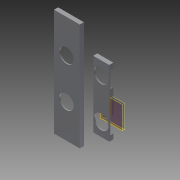
# Autodesk Inventor part: FilterHolder
Saved by Autodesk Inventor 2015 (Build 190159000, 159)
## iProperties
Created: 2015-03-20
Part Number: FilterHolder
Material: NylonD2W
Document SubType Name: Modeling
Designer: Akovo_000
Density: 0.93 g/cm^3
Appearance: Nylon 6
Mass: 9.00848 g
Surface Area: 83.0237 cm^2
Volume: 9.68653 cm^3
Author: Akovo_000
Autodesk Inventor part; units mm, degrees
ref_plane "YZ Plane" through (0, 0, 0) normal (1, 0, 0) x (0, 1, 0)
ref_plane "XZ Plane" through (0, 0, 0) normal (0, 1, 0) x (-1, 0, 0)
ref_plane "Main Work Pane" through (0, 2.75, 7) normal (0, 1, 0) x (-1, 0, 0)
sketch "Panel" plane through (0, 2.75, 7) normal (0, 1, 0) x (-1, 0, 0)
  circle A0 centre (9.0425, 26.1606) radius 11.05 construction
  circle A1 centre (9.0425, -12.8394) radius 11.05 construction
  circle A2 centre (42.8425, -12.8394) radius 11.05
  circle A3 centre (42.8425, 26.1606) radius 11.05
  line L0 (42.8425, -12.8394) -> (42.8425, -12.8394) construction
  line L1 (60.8425, 44.1606) -> (24.8425, 44.1606) construction
  line L2 (24.8425, 44.1606) -> (24.8425, 8.1606) construction
  line L3 (24.8425, 8.1606) -> (60.8425, 8.1606) construction
  line L4 (60.8425, 8.1606) -> (60.8425, 44.1606) construction
  line L5 (60.8425, 44.1606) -> (24.8425, 8.1606) construction
  line L6 (24.8425, 44.1606) -> (60.8425, 8.1606) construction
  line L7 (60.8425, 5.1606) -> (24.8425, 5.1606) construction
  line L8 (24.8425, 5.1606) -> (24.8425, -30.8394) construction
  line L9 (24.8425, -30.8394) -> (60.8425, -30.8394) construction
  line L10 (60.8425, -30.8394) -> (60.8425, 5.1606) construction
  line L11 (60.8425, 5.1606) -> (24.8425, -30.8394) construction
  line L12 (24.8425, 5.1606) -> (60.8425, -30.8394) construction
  line L13 (21.8425, 38.9606) -> (-3.7575, 38.9606) construction
  line L14 (-3.7575, 38.9606) -> (-3.7575, 13.3606) construction
  line L15 (-3.7575, 13.3606) -> (21.8425, 13.3606) construction
  line L16 (21.8425, 13.3606) -> (21.8425, 38.9606) construction
  line L17 (21.8425, 38.9606) -> (-3.7575, 13.3606) construction
  line L18 (-3.7575, 38.9606) -> (21.8425, 13.3606) construction
  line L19 (21.8425, -0.0394) -> (-3.7575, -0.0394) construction
  line L20 (-3.7575, -0.0394) -> (-3.7575, -25.6394) construction
  line L21 (-3.7575, -25.6394) -> (21.8425, -25.6394) construction
  line L22 (21.8425, -25.6394) -> (21.8425, -0.0394) construction
  line L23 (21.8425, -0.0394) -> (-3.7575, -25.6394) construction
  line L24 (-3.7575, -0.0394) -> (21.8425, -25.6394) construction
  line L25 (60.8425, -30.8394) -> (60.8425, 44.1606) construction
  line L26 (60.8425, 44.1606) -> (-3.7575, 44.1606) construction
  line L27 (-3.7575, 44.1606) -> (-3.7575, -30.8394) construction
  line L28 (-3.7575, -30.8394) -> (60.8425, -30.8394) construction
  line L29 (91.5425, -93.8394) -> (-34.4575, -93.8394) construction
  line L30 (-34.4575, -93.8394) -> (-34.4575, 107.1606) construction
  line L31 (-34.4575, 107.1606) -> (91.5425, 107.1606) construction
  line L32 (91.5425, 107.1606) -> (91.5425, -93.8394) construction
  line L33 (42.8425, 15.1106) -> (42.8425, -1.7894) construction
  line L34 (31.7925, 26.1606) -> (20.0925, 26.1606) construction
  line L35 (9.0425, 15.1106) -> (9.0425, -1.7894) construction
  line L36 (20.0925, -12.8394) -> (31.7925, -12.8394) construction
  line L37 (17.4252, 107.1606) -> (17.4252, 44.1606) construction
  line L38 (17.4252, -30.8394) -> (17.4252, -93.8394) construction
  line L39 (60.8425, 6.6606) -> (91.5425, 6.6606) construction
  line L40 (-3.7575, 6.6606) -> (-34.4575, 6.6606) construction
  line L41 (71.3425, 84.9606) -> (89.5425, 84.9606) construction
  line L42 (89.5425, 84.9606) -> (89.5425, 105.1606) construction
  line L43 (89.5425, 105.1606) -> (71.3425, 105.1606) construction
  line L44 (71.3425, 105.1606) -> (71.3425, 84.9606) construction
  line L45 (69.3425, 107.1606) -> (69.3425, 82.9606) construction
  line L46 (69.3425, 82.9606) -> (91.5425, 82.9606) construction
  line L47 (89.5425, -91.8394) -> (71.3425, -91.8394) construction
  line L48 (71.3425, -91.8394) -> (71.3425, -71.6394) construction
  line L49 (71.3425, -71.6394) -> (89.5425, -71.6394) construction
  line L50 (89.5425, -71.6394) -> (89.5425, -91.8394) construction
  line L51 (91.5425, -69.6394) -> (69.3425, -69.6394) construction
  line L52 (69.3425, -69.6394) -> (69.3425, -93.8394) construction
  line L53 (-32.4575, -91.8394) -> (-14.2575, -91.8394) construction
  line L54 (-14.2575, -91.8394) -> (-14.2575, -71.6394) construction
  line L55 (-14.2575, -71.6394) -> (-32.4575, -71.6394) construction
  line L56 (-32.4575, -71.6394) -> (-32.4575, -91.8394) construction
  line L57 (-12.2575, -93.8394) -> (-12.2575, -69.6394) construction
  line L58 (-12.2575, -69.6394) -> (-34.4575, -69.6394) construction
  line L59 (-14.2575, 84.9606) -> (-32.4575, 84.9606) construction
  line L60 (-32.4575, 84.9606) -> (-32.4575, 105.1606) construction
  line L61 (-32.4575, 105.1606) -> (-14.2575, 105.1606) construction
  line L62 (-14.2575, 105.1606) -> (-14.2575, 84.9606) construction
  line L63 (-12.2575, 107.1606) -> (-12.2575, 82.9606) construction
  line L64 (-12.2575, 82.9606) -> (-34.4575, 82.9606) construction
  circle A4 centre (80.4425, 95.0606) radius 2 construction
  line L65 (80.4425, 95.0606) -> (71.3425, 95.0606) construction
  line L66 (80.4425, 95.0606) -> (89.5425, 95.0606) construction
  line L67 (80.4425, 95.0606) -> (80.4425, 105.1606) construction
  line L68 (80.4425, 95.0606) -> (80.4425, 84.9606) construction
  circle A5 centre (-23.3575, 95.0606) radius 2 construction
  line L69 (-23.3575, 95.0606) -> (-23.3575, 84.9606) construction
  line L70 (-23.3575, 95.0606) -> (-23.3575, 105.1606) construction
  line L71 (-23.3575, 95.0606) -> (-32.4575, 95.0606) construction
  line L72 (-23.3575, 95.0606) -> (-14.2575, 95.0606) construction
  circle A6 centre (80.4425, -81.7394) radius 2 construction
  line L73 (80.4425, -81.7394) -> (80.4425, -71.6394) construction
  line L74 (80.4425, -71.6394) -> (80.4425, -81.7394) construction
  line L75 (80.4425, -91.8394) -> (80.4425, -81.7394) construction
  line L76 (80.4425, -81.7394) -> (71.3425, -81.7394) construction
  line L77 (80.4425, -81.7394) -> (89.5425, -81.7394) construction
  circle A7 centre (-23.3575, -81.7394) radius 2 construction
  line L78 (-23.3575, -81.7394) -> (-23.3575, -91.8394) construction
  line L79 (-23.3575, -81.7394) -> (-14.2575, -81.7394) construction
  line L80 (-23.3575, -81.7394) -> (-32.4575, -81.7394) construction
  line L81 (-23.3575, -81.7394) -> (-23.3575, -71.6394) construction
  line L82 (54.9391, 58.7211) -> (29.9084, 58.7211)
  line L83 (29.9084, 58.7211) -> (29.9084, -45.6432)
  line L84 (29.9084, -45.6432) -> (54.9391, -45.6432)
  line L85 (54.9391, -45.6432) -> (54.9391, 58.7211)
  arc A8 (1.229, -20.653) -> (16.856, -20.653) centre (9.0425, -12.8394) ccw
  arc A9 (16.856, -5.0259) -> (1.229, -5.0259) centre (9.0425, -12.8394) ccw
  arc A10 (1.229, 18.347) -> (16.856, 18.347) centre (9.0425, 26.1606) ccw
  arc A11 (16.856, 33.9741) -> (1.229, 33.9741) centre (9.0425, 26.1606) ccw
  line L86 (16.856, -20.653) -> (16.856, -5.0259)
  line L87 (16.856, -5.0259) -> (16.856, 18.347)
  line L88 (16.856, 18.347) -> (16.856, 33.9741)
  line L89 (1.229, 33.9741) -> (1.229, 18.347)
  line L90 (1.229, 18.347) -> (1.229, -5.0259)
  line L91 (1.229, -5.0259) -> (1.229, -20.653)
  line L92 (1.229, -20.653) -> (1.229, -25.6394)
  line L93 (1.229, -25.6394) -> (16.856, -25.6394)
  line L94 (16.856, -25.6394) -> (16.856, -20.653)
  line L95 (16.856, 33.9741) -> (16.856, 38.9606)
  line L96 (16.856, 38.9606) -> (1.229, 38.9606)
  line L97 (1.229, 38.9606) -> (1.229, 33.9741)
  dimension "d337" = 22.1
  dimension "d490" = 36
  dimension "d491" = 36
  dimension "d494" = 3
  dimension "d495" = 25.6
  dimension "d496" = 25.6
  dimension "d497" = 3
  dimension "d498" = 0
  dimension "d582" = 126
  dimension "d583" = 201
  dimension "d584" = 2
  dimension "d585" = 2
  dimension "d586" = 2
  dimension "d587" = 2
  dimension "d588" = 20.2
  dimension "d589" = 18.2
  dimension "d592" = 2
  dimension "d593" = 4
  dimension "d597" = 2
  dimension "d648" = 2
  dimension "d651" = 152.6
  constraints: 196 end point, 27 midpoint, 26 perpendicular, 25 point on line, 23 parallel, 20 equal length, 20 point on circle, 18 collinear, 12 centre point, 11 horizontal, 6 equal radius, 6 line through centre, 6 vertical, 4 coincident
  measures "d337" diameter of A2
  measures "d490" distance of L3.end L2.end
  measures "d491" distance of L2.end L1.end
  measures "d494" distance between parallel lines of L7 L3
  measures "d495" distance of L15.end L14.end
  measures "d496" distance of L14.end L13.end
  measures "d497" distance between parallel lines of L22 L8
  measures "d498" distance between parallel lines of L27 L14
  measures "d582" distance between parallel lines of L30 L32
  measures "d583" distance between parallel lines of L29 L31
  measures "d584" distance between parallel lines of L31 L43
  measures "d585" distance between parallel lines of L32 L42
  measures "d586" distance between parallel lines of L46 L41
  measures "d587" distance between parallel lines of L44 L45
  measures "d588" distance between parallel lines of L41 L43
  measures "d589" distance between parallel lines of L42 L44
  measures "d592" distance between parallel lines of L30 L56
  measures "d593" diameter of A4
  measures "d597" distance between parallel lines of L29 L47
  measures "d648" distance between parallel lines of L62 L63
  measures "d651" distance between parallel lines of L46 L51
ref_plane "Work Plane13" through (0, 2.75, 7) normal (0, -1, 0) x (1, 0, 0)
ref_plane "Work Plane11" through (0, 2.75, 7) normal (0, -1, 0) x (1, 0, 0)
ref_plane "Work Plane12" through (0, 4.75, 7) normal (0, 1, 0) x (1, 0, 0)
extrude "FlatPlane" add sketch "Panel" along normal blind 3 contours L85 L84 L83 L82 | A8 L94 L93 L92 | L90 A10 L87 A9 | L97 L96 L95 A11
sketch "Sketch21" plane through (0, 2.75, 7) normal (0, -1, 0) x (1, 0, 0)
  circle A0 centre (-42.8425, 26.1606) radius 11.05 projected
  circle A1 centre (-42.8425, 26.1606) radius 7
  circle A2 centre (-42.8425, -12.8394) radius 11.05 projected
  circle A3 centre (-42.8425, -12.8394) radius 7
  arc A4 (-1.229, 33.9741) -> (-16.856, 33.9741) centre (-9.0425, 26.1606) ccw projected
  circle A5 centre (-9.0425, 26.1606) radius 7
  arc A6 (-16.856, -20.653) -> (-1.229, -20.653) centre (-9.0425, -12.8394) ccw projected
  circle A7 centre (-9.0425, -12.8394) radius 7
  line L0 (-54.9391, 58.7211) -> (-29.9084, 58.7211)
  line L1 (-29.9084, 58.7211) -> (-29.9084, -45.6432)
  line L2 (-29.9084, -45.6432) -> (-54.9391, -45.6432)
  line L3 (-54.9391, -45.6432) -> (-54.9391, 58.7211)
  line L4 (-16.856, 38.9606) -> (-1.229, 38.9606)
  line L5 (-1.229, 38.9606) -> (-1.229, -25.6394)
  line L6 (-1.229, -25.6394) -> (-16.856, -25.6394)
  line L7 (-16.856, -25.6394) -> (-16.856, 38.9606)
  point P0 (0, -7)
  dimension "d656" = 14
  constraints: 16 end point, 4 centre point, 4 coincident, 4 parallel, 3 equal radius, 2 horizontal, 2 perpendicular
  measures "d656" diameter of A1
extrude "Extrusion18" add sketch "Sketch21" along normal blind 1 contours A0 | A2 | L5 A6 L7 A4 | A4 L7 L4 L5 | L5 L6 L7 A6 | L0 L1 L2 L3
body "Solid3"
